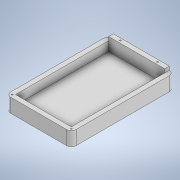
# Autodesk Inventor part: CARCASA SUPERIOR
Saved by Autodesk Inventor 2020 (Build 240168000, 168)
## iProperties
Created: 2022-05-22
Part Number: CARCASA SUPERIOR
Material: Generic
Document SubType Name: Modeling
Designer: juanc
Density: 1 g/cm^3
Appearance: Default
Author: juanc
## iProperties of the stored document _3DPrint.ipt
Created: 2022-05-23
Part Number: _3DPrint
Material: Generic
Document SubType Name: Modeling
Designer: juanc
Density: 1 g/cm^3
Appearance: Default
Author: juanc
Autodesk Inventor part; units mm, degrees
ref_plane "YZ Plane" through (0, 0, 0) normal (1, 0, 0) x (0, 1, 0)
ref_plane "XZ Plane" through (0, 0, 0) normal (0, 1, 0) x (-1, 0, 0)
ref_plane "XY Plane" through (0, 0, 0) normal (0, 0, 1) x (1, 0, 0)
sketch "Sketch1" plane through (0, 0, 0) normal (0, 1, 0) x (-1, 0, 0)
  line L0 (0, 0) -> (70, 0)
  line L1 (70, 0) -> (70, -110)
  line L2 (70, -110) -> (0, -110)
  line L3 (0, -110) -> (0, 0)
  line L4 (70, 0) -> (0, -110) construction
  line L5 (70, -110) -> (0, 0) construction
  line L6 (65, -5) -> (5, -5)
  line L7 (5, -5) -> (5, -105)
  line L8 (5, -105) -> (65, -105)
  line L9 (65, -105) -> (65, -5)
  line L10 (65, -5) -> (5, -105) construction
  line L11 (5, -5) -> (65, -105) construction
  point P0 (35, -55)
  dimension "d0" = 70
  dimension "d1" = 110
  dimension "d2" = 60
  dimension "d3" = 100
  constraints: 24 end point, 4 parallel, 3 midpoint, 2 horizontal, 2 perpendicular
  measures "d0" distance of L1.end L2.end
  measures "d1" distance of L0.end L1.end
  measures "d2" distance of L8.end L7.end
  measures "d3" distance of L7.end L6.end
extrude "Extrusion1" add sketch "Sketch1" along normal blind 15
extrude "Extrusion2" add sketch "Sketch1" along normal blind 5 contours L9 L8 L7 L6
fillet "Fillet1" radius 5 4 edges at (0, 7.5, -110) (0, 7.5, 0) (-70, 7.5, 0) (-70, 7.5, -110)
sketch "Sketch2" plane through (-5, 0, -110) normal (0, 0, -1) x (-1, 0, 0)
  line L0 (0, 15) -> (60, 15) projected
  line L1 (60, 15) -> (0, 15)
  line L2 (0, 15) -> (0, 19)
  line L3 (0, 19) -> (60, 19)
  line L4 (60, 19) -> (60, 15)
  point P0 (-5, 0)
  dimension "d9" = 60
  dimension "d10" = 4
  constraints: 8 end point, 2 parallel, 1 horizontal, 1 perpendicular
  measures "d9" distance of L2.end L3.end
  measures "d10" distance of L1.end L2.end
extrude "Extrusion3" add sketch "Sketch2" against normal blind 5
sketch "Sketch3" plane through (0, 0, 0) normal (0, -1, 0) x (1, 0, 0)
  arc A0 (-65, 0) -> (-70, -5) centre (-65, -5) ccw construction
  line L0 (-65, -5) -> (-66.7678, -3.2322) construction
  line L1 (-65, -5) -> (-62.5, -5) construction
  arc A1 (0, -5) -> (-5, 0) centre (-5, -5) ccw construction
  line L2 (-5, -5) -> (-3.2322, -3.2322) construction
  point P0 (0, 0)
  dimension "d13" = 2.5
  dimension "d14" = 135
  dimension "d15" = 2.5
  constraints: 6 end point, 2 coincident, 1 equal length, 1 horizontal
  measures "d13" distance of L0.start L0.end
  measures "d14" angle of L1 L0
  measures "d15" distance of L2.start L2.end
hole "Hole1" at (-66.7678, 0, -3.2322) at (-3.2322, 0, -3.2322) direction (0, 1, 0) diameter 1.5 depth 40 tip angle 118 counterbore diameter 2.5 counterbore depth 1
sketch "Sketch4" plane through (0, 0, 0) normal (0, -1, 0) x (1, 0, 0)
  line L0 (-65, -105) -> (-65, -110) construction
  line L1 (-5, -110) -> (-5, -105) construction
  line L2 (-5, -105) -> (-5, -5) construction
  line L3 (-5, -110) -> (-5, -105) construction
  line L4 (-5, -110) -> (-65, -110) construction
  line L5 (-35, -107.5) -> (-5, -107.5) construction
  line L6 (-35, -107.5) -> (-65, -107.5) construction
  line L7 (-35, -107.5) -> (-15, -107.5) construction
  line L8 (-35, -107.5) -> (-15, -107.5) construction
  line L9 (-35, -107.5) -> (-55, -107.5) construction
  line L10 (-35, -107.5) -> (-15, -107.5) construction
  point P0 (0, 0)
  dimension "d23" = 20
  dimension "d24" = 0
  dimension "d25" = 20
  dimension "d26" = 180
  constraints: 14 end point, 4 collinear, 2 coincident, 2 horizontal, 2 midpoint
  measures "d23" distance of L5.start L7.end
  measures "d24" distance between parallel lines of L7 L8
  measures "d25" distance of L5.start L9.end
  measures "d26" angle of L9 L10
hole "Hole2" at (-55, 0, -107.5) at (-15, 0, -107.5) direction (0, 1, 0) diameter 1.5 depth 40 tip angle 118 counterbore diameter 2.5 counterbore depth 1
sketch "Sketch5" plane through (0, 0, 0) normal (0, -1, 0) x (1, 0, 0)
  line L0 (-19.9406, -8.9451) -> (-19.9406, -100.011) construction
  line L1 (-19.9406, -100.011) -> (-26.1694, -100.011) construction
  line L2 (-26.1694, -100.011) -> (-26.1694, -8.9451) construction
  line L3 (-26.1694, -8.9451) -> (-19.9406, -8.9451) construction
  line L4 (-53.1117, -60.5446) -> (-53.1117, -96.1252) construction
  line L5 (-53.1117, -96.1252) -> (-61.1378, -96.1252) construction
  line L6 (-61.1378, -96.1252) -> (-61.1378, -60.5446) construction
  line L7 (-61.1378, -60.5446) -> (-53.1117, -60.5446) construction
  line L8 (-23.7466, -10.3806) -> (-26.0645, -10.3806)
  line L9 (-26.0645, -10.3806) -> (-26.0645, -9.5603)
  line L10 (-26.0645, -9.5603) -> (-20.0503, -9.5603)
  spline S0 degree 2 poles (-20.0503, -9.5603) (-20.0074, -10.4951) (-20.0074, -10.6859) knots 0 0 0 1 1 1
  spline S1 degree 2 poles (-20.0074, -10.6859) (-20.0074, -13.309) (-21.7625, -13.309) knots 0 0 0 1 1 1
  spline S2 degree 2 poles (-21.7625, -13.309) (-23.7895, -13.309) (-23.7895, -10.9911) knots 0 0 0 1 1 1
  spline S3 degree 2 poles (-23.7895, -10.9911) (-23.7895, -10.848) (-23.7466, -10.3806) knots 0 0 0 1 1 1
  line L11 (-20.7896, -10.3806) -> (-23.0073, -10.3806)
  spline S4 degree 2 poles (-23.0073, -10.3806) (-23.0502, -10.9053) (-23.0502, -10.9339) knots 0 0 0 1 1 1
  spline S5 degree 2 poles (-23.0502, -10.9339) (-23.0502, -12.4648) (-21.8484, -12.4648) knots 0 0 0 1 1 1
  spline S6 degree 2 poles (-21.8484, -12.4648) (-20.7466, -12.4648) (-20.7466, -10.829) knots 0 0 0 1 1 1
  spline S7 degree 2 poles (-20.7466, -10.829) (-20.7466, -10.6668) (-20.7896, -10.3806) knots 0 0 0 1 1 1
  line L12 (-26.0645, -17.5967) -> (-23.4795, -15.9894)
  spline S8 degree 2 poles (-23.4795, -15.9894) (-23.4795, -15.7128) (-23.4366, -15.1166) knots 0 0 0 1 1 1
  line L13 (-23.4366, -15.1166) -> (-26.0645, -15.1166)
  line L14 (-26.0645, -15.1166) -> (-26.0645, -14.2963)
  line L15 (-26.0645, -14.2963) -> (-20.0455, -14.2963)
  spline S9 degree 2 poles (-20.0455, -14.2963) (-20.0455, -14.3392) (-19.9835, -15.5268) (-19.9835, -15.7986) knots 0 0 0 1 2 2 2
  spline S10 degree 2 poles (-19.9835, -15.7986) (-19.9835, -17.9687) (-21.71, -17.9687) knots 0 0 0 1 1 1
  spline S11 degree 2 poles (-21.71, -17.9687) (-22.2776, -17.9687) (-23.1838, -17.2723) (-23.2935, -16.7906) knots 0 0 0 1 2 2 2
  line L16 (-23.2935, -16.7906) -> (-26.0645, -18.5362)
  line L17 (-26.0645, -18.5362) -> (-26.0645, -17.5967)
  line L18 (-20.7848, -15.1166) -> (-22.7402, -15.1166)
  spline S12 degree 2 poles (-22.7402, -15.1166) (-22.7831, -15.4123) (-22.7831, -15.6937) knots 0 0 0 1 1 1
  spline S13 degree 2 poles (-22.7831, -15.6937) (-22.7831, -16.4329) (-22.3062, -17.1054) (-21.691, -17.1054) knots 0 0 0 1 2 2 2
  spline S14 degree 2 poles (-21.691, -17.1054) (-21.1854, -17.1054) (-20.7419, -16.3805) (-20.7419, -15.6031) knots 0 0 0 1 2 2 2
  spline S15 degree 2 poles (-20.7419, -15.6031) (-20.7419, -15.4791) (-20.7848, -15.1166) knots 0 0 0 1 1 1
  spline S16 degree 2 poles (-23.0073, -18.8653) (-21.7005, -18.8653) (-19.9406, -20.1769) (-19.9406, -21.2881) knots 0 0 0 1 2 2 2
  spline S17 degree 2 poles (-19.9406, -21.2881) (-19.9406, -22.5425) (-21.5574, -23.8779) (-23.0073, -23.8779) knots 0 0 0 1 2 2 2
  spline S18 degree 2 poles (-23.0073, -23.8779) (-24.4906, -23.8779) (-26.1694, -22.5377) (-26.1694, -21.2881) knots 0 0 0 1 2 2 2
  spline S19 degree 2 poles (-26.1694, -21.2881) (-26.1694, -20.153) (-24.3952, -18.8653) (-23.0073, -18.8653) knots 0 0 0 1 2 2 2
  spline S20 degree 2 poles (-23.0073, -19.7286) (-24.0423, -19.7286) (-25.4301, -20.5441) (-25.4301, -21.2881) knots 0 0 0 1 2 2 2
  spline S21 degree 2 poles (-25.4301, -21.2881) (-25.4301, -22.1323) (-24.1567, -23.0146) (-23.0073, -23.0146) knots 0 0 0 1 2 2 2
  spline S22 degree 2 poles (-23.0073, -23.0146) (-20.6799, -23.0146) (-20.6799, -21.2881) knots 0 0 0 1 1 1
  spline S23 degree 2 poles (-20.6799, -21.2881) (-20.6799, -20.525) (-21.9294, -19.7286) (-23.0073, -19.7286) knots 0 0 0 1 2 2 2
  line L19 (-23.3698, -27.0209) -> (-26.0645, -27.0209)
  line L20 (-26.0645, -27.0209) -> (-26.0645, -26.2006)
  line L21 (-26.0645, -26.2006) -> (-23.3698, -26.2006)
  line L22 (-23.3698, -26.2006) -> (-20.0455, -24.2594)
  line L23 (-20.0455, -24.2594) -> (-20.0455, -25.1036)
  line L24 (-20.0455, -25.1036) -> (-22.6735, -26.606)
  line L25 (-22.6735, -26.606) -> (-20.0455, -28.1083)
  line L26 (-20.0455, -28.1083) -> (-20.0455, -28.9525)
  line L27 (-20.0455, -28.9525) -> (-23.3698, -27.0209)
  line L28 (-20.7848, -30.4405) -> (-22.4588, -30.4405)
  line L29 (-22.4588, -30.4405) -> (-22.4588, -32.3864)
  line L30 (-22.4588, -32.3864) -> (-23.1552, -32.3864)
  line L31 (-23.1552, -32.3864) -> (-23.1552, -30.4405)
  line L32 (-23.1552, -30.4405) -> (-25.3252, -30.4405)
  line L33 (-25.3252, -30.4405) -> (-25.3252, -33.1734)
  line L34 (-25.3252, -33.1734) -> (-26.0645, -33.1734)
  line L35 (-26.0645, -33.1734) -> (-26.0645, -29.6202)
  line L36 (-26.0645, -29.6202) -> (-20.0455, -29.6202)
  line L37 (-20.0455, -29.6202) -> (-20.0455, -33.1734)
  line L38 (-20.0455, -33.1734) -> (-20.7848, -33.1734)
  line L39 (-20.7848, -33.1734) -> (-20.7848, -30.4405)
  line L40 (-20.2697, -37.9666) -> (-20.9708, -37.6899)
  spline S24 degree 2 poles (-20.9708, -37.6899) (-20.6846, -37.2989) (-20.6846, -36.4547) knots 0 0 0 1 1 1
  spline S25 degree 2 poles (-20.6846, -36.4547) (-20.6846, -35.6582) (-22.0487, -34.7043) (-23.1265, -34.7043) knots 0 0 0 1 2 2 2
  spline S26 degree 2 poles (-23.1265, -34.7043) (-24.152, -34.7043) (-25.4301, -35.6868) (-25.4301, -36.4594) knots 0 0 0 1 2 2 2
  spline S27 degree 2 poles (-25.4301, -36.4594) (-25.4301, -37.3084) (-24.8292, -37.7615) knots 0 0 0 1 1 1
  line L41 (-24.8292, -37.7615) -> (-25.4588, -38.2146)
  spline S28 degree 2 poles (-25.4588, -38.2146) (-26.1694, -37.4992) (-26.1694, -36.3736) knots 0 0 0 1 1 1
  spline S29 degree 2 poles (-26.1694, -36.3736) (-26.1694, -35.1956) (-24.4667, -33.8411) (-23.0741, -33.8411) knots 0 0 0 1 2 2 2
  spline S30 degree 2 poles (-23.0741, -33.8411) (-21.7291, -33.8411) (-19.9454, -35.2862) (-19.9454, -36.4308) knots 0 0 0 1 2 2 2
  spline S31 degree 2 poles (-19.9454, -36.4308) (-19.9454, -37.4133) (-20.2697, -37.9666) knots 0 0 0 1 1 1
  line L42 (-20.7848, -41.3528) -> (-26.0645, -41.3528)
  line L43 (-26.0645, -41.3528) -> (-26.0645, -40.5325)
  line L44 (-26.0645, -40.5325) -> (-20.7848, -40.5325)
  line L45 (-20.7848, -40.5325) -> (-20.7848, -38.62)
  line L46 (-20.7848, -38.62) -> (-20.0455, -38.62)
  line L47 (-20.0455, -38.62) -> (-20.0455, -43.3512)
  line L48 (-20.0455, -43.3512) -> (-20.7848, -43.3512)
  line L49 (-20.7848, -43.3512) -> (-20.7848, -41.3528)
  spline S32 degree 2 poles (-23.0073, -43.7566) (-21.7005, -43.7566) (-19.9406, -45.0681) (-19.9406, -46.1794) knots 0 0 0 1 2 2 2
  spline S33 degree 2 poles (-19.9406, -46.1794) (-19.9406, -47.4337) (-21.5574, -48.7691) (-23.0073, -48.7691) knots 0 0 0 1 2 2 2
  spline S34 degree 2 poles (-23.0073, -48.7691) (-24.4906, -48.7691) (-26.1694, -47.429) (-26.1694, -46.1794) knots 0 0 0 1 2 2 2
  spline S35 degree 2 poles (-26.1694, -46.1794) (-26.1694, -45.0443) (-24.3952, -43.7566) (-23.0073, -43.7566) knots 0 0 0 1 2 2 2
  spline S36 degree 2 poles (-23.0073, -44.6198) (-24.0423, -44.6198) (-25.4301, -45.4354) (-25.4301, -46.1794) knots 0 0 0 1 2 2 2
  spline S37 degree 2 poles (-25.4301, -46.1794) (-25.4301, -47.0236) (-24.1567, -47.9059) (-23.0073, -47.9059) knots 0 0 0 1 2 2 2
  spline S38 degree 2 poles (-23.0073, -47.9059) (-20.6799, -47.9059) (-20.6799, -46.1794) knots 0 0 0 1 1 1
  spline S39 degree 2 poles (-20.6799, -46.1794) (-20.6799, -45.4163) (-21.9294, -44.6198) (-23.0073, -44.6198) knots 0 0 0 1 2 2 2
  line L50 (-26.0645, -52.3891) -> (-20.0455, -52.3891)
  line L51 (-20.0455, -52.3891) -> (-20.0455, -53.2094)
  line L52 (-20.0455, -53.2094) -> (-26.0645, -53.2094)
  line L53 (-26.0645, -53.2094) -> (-26.0645, -52.3891)
  line L54 (-26.1455, -58.4795) -> (-21.7482, -55.3699)
  line L55 (-21.7482, -55.3699) -> (-26.0645, -55.3699)
  line L56 (-26.0645, -55.3699) -> (-26.0645, -54.5877)
  line L57 (-26.0645, -54.5877) -> (-20.0455, -54.5877)
  line L58 (-20.0455, -54.5877) -> (-20.0455, -54.9168)
  line L59 (-20.0455, -54.9168) -> (-24.2044, -57.9454)
  line L60 (-24.2044, -57.9454) -> (-20.0455, -57.9454)
  line L61 (-20.0455, -57.9454) -> (-20.0455, -58.7275)
  line L62 (-20.0455, -58.7275) -> (-26.1455, -58.7275)
  line L63 (-26.1455, -58.7275) -> (-26.1455, -58.4795)
  line L64 (-20.7848, -62.1519) -> (-26.0645, -62.1519)
  line L65 (-26.0645, -62.1519) -> (-26.0645, -61.3316)
  line L66 (-26.0645, -61.3316) -> (-20.7848, -61.3316)
  line L67 (-20.7848, -61.3316) -> (-20.7848, -59.4191)
  line L68 (-20.7848, -59.4191) -> (-20.0455, -59.4191)
  line L69 (-20.0455, -59.4191) -> (-20.0455, -64.1503)
  line L70 (-20.0455, -64.1503) -> (-20.7848, -64.1503)
  line L71 (-20.7848, -64.1503) -> (-20.7848, -62.1519)
  line L72 (-20.7848, -65.6622) -> (-22.4588, -65.6622)
  line L73 (-22.4588, -65.6622) -> (-22.4588, -67.6081)
  line L74 (-22.4588, -67.6081) -> (-23.1552, -67.6081)
  line L75 (-23.1552, -67.6081) -> (-23.1552, -65.6622)
  line L76 (-23.1552, -65.6622) -> (-25.3252, -65.6622)
  line L77 (-25.3252, -65.6622) -> (-25.3252, -68.395)
  line L78 (-25.3252, -68.395) -> (-26.0645, -68.395)
  line L79 (-26.0645, -68.395) -> (-26.0645, -64.8419)
  line L80 (-26.0645, -64.8419) -> (-20.0455, -64.8419)
  line L81 (-20.0455, -64.8419) -> (-20.0455, -68.395)
  line L82 (-20.0455, -68.395) -> (-20.7848, -68.395)
  line L83 (-20.7848, -68.395) -> (-20.7848, -65.6622)
  line L84 (-20.4652, -73.5221) -> (-21.1425, -73.1787)
  spline S40 degree 2 poles (-21.1425, -73.1787) (-20.6846, -72.5587) (-20.6846, -71.9625) knots 0 0 0 1 1 1
  spline S41 degree 2 poles (-20.6846, -71.9625) (-20.6846, -71.0182) (-22.0153, -69.926) (-23.1122, -69.926) knots 0 0 0 1 2 2 2
  spline S42 degree 2 poles (-23.1122, -69.926) (-24.1567, -69.926) (-25.4301, -70.9991) (-25.4301, -71.9243) knots 0 0 0 1 2 2 2
  spline S43 degree 2 poles (-25.4301, -71.9243) (-25.4301, -72.5825) (-25.0343, -72.9879) knots 0 0 0 1 1 1
  line L85 (-25.0343, -72.9879) -> (-23.6226, -72.9879)
  line L86 (-23.6226, -72.9879) -> (-23.6226, -72.1533)
  line L87 (-23.6226, -72.1533) -> (-22.9262, -72.1533)
  line L88 (-22.9262, -72.1533) -> (-22.9262, -73.8082)
  line L89 (-22.9262, -73.8082) -> (-25.5494, -73.8082)
  spline S44 degree 2 poles (-25.5494, -73.8082) (-25.826, -73.4791) (-26.1694, -72.3059) (-26.1694, -71.7479) knots 0 0 0 1 2 2 2
  spline S45 degree 2 poles (-26.1694, -71.7479) (-26.1694, -70.5031) (-24.481, -69.0627) (-23.0788, -69.0627) knots 0 0 0 1 2 2 2
  spline S46 degree 2 poles (-23.0788, -69.0627) (-21.6814, -69.0627) (-19.9454, -70.6462) (-19.9454, -71.9911) knots 0 0 0 1 2 2 2
  spline S47 degree 2 poles (-19.9454, -71.9911) (-19.9454, -72.9307) (-20.4652, -73.5221) knots 0 0 0 1 1 1
  line L90 (-26.0645, -78.382) -> (-23.4795, -76.7748)
  spline S48 degree 2 poles (-23.4795, -76.7748) (-23.4795, -76.4981) (-23.4366, -75.902) knots 0 0 0 1 1 1
  line L91 (-23.4366, -75.902) -> (-26.0645, -75.902)
  line L92 (-26.0645, -75.902) -> (-26.0645, -75.0817)
  line L93 (-26.0645, -75.0817) -> (-20.0455, -75.0817)
  spline S49 degree 2 poles (-20.0455, -75.0817) (-20.0455, -75.1246) (-19.9835, -76.3121) (-19.9835, -76.584) knots 0 0 0 1 2 2 2
  spline S50 degree 2 poles (-19.9835, -76.584) (-19.9835, -78.7541) (-21.71, -78.7541) knots 0 0 0 1 1 1
  spline S51 degree 2 poles (-21.71, -78.7541) (-22.2776, -78.7541) (-23.1838, -78.0577) (-23.2935, -77.576) knots 0 0 0 1 2 2 2
  line L94 (-23.2935, -77.576) -> (-26.0645, -79.3216)
  line L95 (-26.0645, -79.3216) -> (-26.0645, -78.382)
  line L96 (-20.7848, -75.902) -> (-22.7402, -75.902)
  spline S52 degree 2 poles (-22.7402, -75.902) (-22.7831, -76.1977) (-22.7831, -76.4791) knots 0 0 0 1 1 1
  spline S53 degree 2 poles (-22.7831, -76.4791) (-22.7831, -77.2183) (-22.3062, -77.8908) (-21.691, -77.8908) knots 0 0 0 1 2 2 2
  spline S54 degree 2 poles (-21.691, -77.8908) (-21.1854, -77.8908) (-20.7419, -77.1659) (-20.7419, -76.3885) knots 0 0 0 1 2 2 2
  spline S55 degree 2 poles (-20.7419, -76.3885) (-20.7419, -76.2645) (-20.7848, -75.902) knots 0 0 0 1 1 1
  line L97 (-26.0645, -83.3565) -> (-24.7958, -82.9415)
  line L98 (-24.7958, -82.9415) -> (-24.7958, -80.7047)
  line L99 (-24.7958, -80.7047) -> (-26.0645, -80.2612)
  line L100 (-26.0645, -80.2612) -> (-26.0645, -79.3407)
  line L101 (-26.0645, -79.3407) -> (-19.9645, -81.7826)
  line L102 (-19.9645, -81.7826) -> (-19.9645, -82.002)
  line L103 (-19.9645, -82.002) -> (-26.0645, -84.2674)
  line L104 (-26.0645, -84.2674) -> (-26.0645, -83.3565)
  line L105 (-21.5431, -81.8541) -> (-24.1901, -80.9241)
  line L106 (-24.1901, -80.9241) -> (-24.1901, -82.7078)
  line L107 (-24.1901, -82.7078) -> (-21.5431, -81.8541)
  line L108 (-26.0645, -86.1084) -> (-26.0645, -84.897)
  line L109 (-26.0645, -84.897) -> (-20.0503, -84.897)
  spline S56 degree 2 poles (-20.0503, -84.897) (-20.0074, -86.0559) (-20.0074, -86.3802) knots 0 0 0 1 1 1
  spline S57 degree 2 poles (-20.0074, -86.3802) (-20.0074, -87.6394) (-21.5383, -89.1083) (-22.8118, -89.1083) knots 0 0 0 1 2 2 2
  spline S58 degree 2 poles (-22.8118, -89.1083) (-26.0645, -89.1083) (-26.0645, -86.1084) knots 0 0 0 1 1 1
  line L110 (-20.7896, -85.7173) -> (-25.2823, -85.7173)
  spline S59 degree 2 poles (-25.2823, -85.7173) (-25.3252, -85.9939) (-25.3252, -86.3993) knots 0 0 0 1 1 1
  spline S60 degree 2 poles (-25.3252, -86.3993) (-25.3252, -87.2626) (-24.0327, -88.2451) (-22.8833, -88.2451) knots 0 0 0 1 2 2 2
  spline S61 degree 2 poles (-22.8833, -88.2451) (-20.7466, -88.2451) (-20.7466, -86.3278) knots 0 0 0 1 1 1
  spline S62 degree 2 poles (-20.7466, -86.3278) (-20.7466, -86.2133) (-20.7896, -85.7173) knots 0 0 0 1 1 1
  spline S63 degree 2 poles (-23.0073, -89.7713) (-21.7005, -89.7713) (-19.9406, -91.0828) (-19.9406, -92.1941) knots 0 0 0 1 2 2 2
  spline S64 degree 2 poles (-19.9406, -92.1941) (-19.9406, -93.4484) (-21.5574, -94.7838) (-23.0073, -94.7838) knots 0 0 0 1 2 2 2
  spline S65 degree 2 poles (-23.0073, -94.7838) (-24.4906, -94.7838) (-26.1694, -93.4437) (-26.1694, -92.1941) knots 0 0 0 1 2 2 2
  spline S66 degree 2 poles (-26.1694, -92.1941) (-26.1694, -91.059) (-24.3952, -89.7713) (-23.0073, -89.7713) knots 0 0 0 1 2 2 2
  spline S67 degree 2 poles (-23.0073, -90.6345) (-24.0423, -90.6345) (-25.4301, -91.4501) (-25.4301, -92.1941) knots 0 0 0 1 2 2 2
  spline S68 degree 2 poles (-25.4301, -92.1941) (-25.4301, -93.0383) (-24.1567, -93.9206) (-23.0073, -93.9206) knots 0 0 0 1 2 2 2
  spline S69 degree 2 poles (-23.0073, -93.9206) (-20.6799, -93.9206) (-20.6799, -92.1941) knots 0 0 0 1 1 1
  spline S70 degree 2 poles (-20.6799, -92.1941) (-20.6799, -91.431) (-21.9294, -90.6345) (-23.0073, -90.6345) knots 0 0 0 1 2 2 2
  line L111 (-26.0645, -99.0715) -> (-23.4795, -97.4642)
  spline S71 degree 2 poles (-23.4795, -97.4642) (-23.4795, -97.1876) (-23.4366, -96.5914) knots 0 0 0 1 1 1
  line L112 (-23.4366, -96.5914) -> (-26.0645, -96.5914)
  line L113 (-26.0645, -96.5914) -> (-26.0645, -95.7711)
  line L114 (-26.0645, -95.7711) -> (-20.0455, -95.7711)
  spline S72 degree 2 poles (-20.0455, -95.7711) (-20.0455, -95.814) (-19.9835, -97.0016) (-19.9835, -97.2734) knots 0 0 0 1 2 2 2
  spline S73 degree 2 poles (-19.9835, -97.2734) (-19.9835, -99.4435) (-21.71, -99.4435) knots 0 0 0 1 1 1
  spline S74 degree 2 poles (-21.71, -99.4435) (-22.2776, -99.4435) (-23.1838, -98.7472) (-23.2935, -98.2655) knots 0 0 0 1 2 2 2
  line L115 (-23.2935, -98.2655) -> (-26.0645, -100.011)
  line L116 (-26.0645, -100.011) -> (-26.0645, -99.0715)
  line L117 (-20.7848, -96.5914) -> (-22.7402, -96.5914)
  spline S75 degree 2 poles (-22.7402, -96.5914) (-22.7831, -96.8871) (-22.7831, -97.1685) knots 0 0 0 1 1 1
  spline S76 degree 2 poles (-22.7831, -97.1685) (-22.7831, -97.9078) (-22.3062, -98.5802) (-21.691, -98.5802) knots 0 0 0 1 2 2 2
  spline S77 degree 2 poles (-21.691, -98.5802) (-21.1854, -98.5802) (-20.7419, -97.8553) (-20.7419, -97.0779) knots 0 0 0 1 2 2 2
  spline S78 degree 2 poles (-20.7419, -97.0779) (-20.7419, -96.9539) (-20.7848, -96.5914) knots 0 0 0 1 1 1
  line L118 (-56.224, -63.0344) -> (-56.224, -62.5799)
  line L119 (-56.224, -62.5799) -> (-53.5959, -61.2313)
  line L120 (-53.5959, -61.2313) -> (-56.224, -61.2313)
  line L121 (-56.224, -61.2313) -> (-56.224, -60.8533)
  line L122 (-56.224, -60.8533) -> (-53.176, -60.8533)
  line L123 (-53.176, -60.8533) -> (-53.176, -61.4289)
  line L124 (-53.176, -61.4289) -> (-55.5892, -62.6565)
  line L125 (-55.5892, -62.6565) -> (-53.176, -62.6565)
  line L126 (-53.176, -62.6565) -> (-53.176, -63.0344)
  line L127 (-53.176, -63.0344) -> (-56.224, -63.0344)
  spline S79 degree 2 poles (-53.5242, -65.8082) (-53.7268, -65.9811) (-54.3196, -66.1738) (-54.7, -66.1738) knots 0 0 0 1 2 2 2
  spline S80 degree 2 poles (-54.7, -66.1738) (-55.0705, -66.1738) (-55.6707, -65.986) (-55.8732, -65.8082) knots 0 0 0 1 2 2 2
  spline S81 degree 2 poles (-55.8732, -65.8082) (-56.0856, -65.6205) (-56.2882, -65.124) (-56.2882, -64.8251) knots 0 0 0 1 2 2 2
  spline S82 degree 2 poles (-56.2882, -64.8251) (-56.2882, -64.5164) (-56.0782, -64.0224) (-55.8732, -63.8421) knots 0 0 0 1 2 2 2
  spline S83 degree 2 poles (-55.8732, -63.8421) (-55.6707, -63.6667) (-55.0754, -63.479) (-54.7, -63.479) knots 0 0 0 1 2 2 2
  spline S84 degree 2 poles (-54.7, -63.479) (-54.3171, -63.479) (-53.7342, -63.6692) (-53.5242, -63.8445) knots 0 0 0 1 2 2 2
  spline S85 degree 2 poles (-53.5242, -63.8445) (-53.3217, -64.0224) (-53.1117, -64.5189) (-53.1117, -64.8251) knots 0 0 0 1 2 2 2
  spline S86 degree 2 poles (-53.1117, -64.8251) (-53.1117, -65.1364) (-53.3291, -65.6353) (-53.5242, -65.8082) knots 0 0 0 1 2 2 2
  spline S87 degree 2 poles (-54.7, -65.7514) (-54.3986, -65.7514) (-53.9318, -65.6205) (-53.7786, -65.5019) knots 0 0 0 1 2 2 2
  spline S88 degree 2 poles (-53.7786, -65.5019) (-53.6206, -65.3809) (-53.4625, -65.04) (-53.4625, -64.8276) knots 0 0 0 1 2 2 2
  spline S89 degree 2 poles (-53.4625, -64.8276) (-53.4625, -64.6078) (-53.6156, -64.2768) (-53.7786, -64.1508) knots 0 0 0 1 2 2 2
  spline S90 degree 2 poles (-53.7786, -64.1508) (-53.9343, -64.0298) (-54.4036, -63.9013) (-54.7, -63.9013) knots 0 0 0 1 2 2 2
  spline S91 degree 2 poles (-54.7, -63.9013) (-55.3002, -63.9013) (-55.9374, -64.4052) (-55.9374, -64.8276) knots 0 0 0 1 2 2 2
  spline S92 degree 2 poles (-55.9374, -64.8276) (-55.9374, -65.25) (-55.3002, -65.7514) (-54.7, -65.7514) knots 0 0 0 1 2 2 2
  line L128 (-53.176, -68.7525) -> (-54.8753, -67.7225)
  line L129 (-54.8753, -67.7225) -> (-56.224, -67.7225)
  line L130 (-56.224, -67.7225) -> (-56.224, -67.3174)
  line L131 (-56.224, -67.3174) -> (-54.9173, -67.3174)
  line L132 (-54.9173, -67.3174) -> (-53.176, -66.2874)
  line L133 (-53.176, -66.2874) -> (-53.176, -66.7369)
  line L134 (-53.176, -66.7369) -> (-54.5172, -67.5224)
  line L135 (-54.5172, -67.5224) -> (-53.176, -68.3227)
  line L136 (-53.176, -68.3227) -> (-53.176, -68.7525)
  line L137 (-56.224, -68.7055) -> (-53.176, -69.7331)
  line L138 (-53.176, -69.7331) -> (-53.176, -70.232)
  line L139 (-53.176, -70.232) -> (-56.224, -71.2595)
  line L140 (-56.224, -71.2595) -> (-56.224, -70.8322)
  line L141 (-56.224, -70.8322) -> (-55.3718, -70.5556)
  line L142 (-55.3718, -70.5556) -> (-55.3718, -69.3922)
  line L143 (-55.3718, -69.3922) -> (-56.224, -69.1156)
  line L144 (-56.224, -69.1156) -> (-56.224, -68.7055)
  line L145 (-55.026, -70.4444) -> (-53.5909, -69.9726)
  line L146 (-53.5909, -69.9726) -> (-55.026, -69.5033)
  line L147 (-55.026, -69.5033) -> (-55.026, -70.4444)
  line L148 (-55.0754, -73.8876) -> (-55.0754, -72.7341)
  line L149 (-55.0754, -72.7341) -> (-54.7049, -72.7341)
  line L150 (-54.7049, -72.7341) -> (-54.7049, -73.8876)
  line L151 (-54.7049, -73.8876) -> (-55.0754, -73.8876)
  line L152 (-56.224, -75.3598) -> (-53.176, -76.3873)
  line L153 (-53.176, -76.3873) -> (-53.176, -76.8862)
  line L154 (-53.176, -76.8862) -> (-56.224, -77.9137)
  line L155 (-56.224, -77.9137) -> (-56.224, -77.4864)
  line L156 (-56.224, -77.4864) -> (-55.3718, -77.2098)
  line L157 (-55.3718, -77.2098) -> (-55.3718, -76.0464)
  line L158 (-55.3718, -76.0464) -> (-56.224, -75.7698)
  line L159 (-56.224, -75.7698) -> (-56.224, -75.3598)
  line L160 (-55.026, -77.0986) -> (-53.5909, -76.6269)
  line L161 (-53.5909, -76.6269) -> (-55.026, -76.1576)
  line L162 (-55.026, -76.1576) -> (-55.026, -77.0986)
  line L163 (-56.224, -79.9688) -> (-56.224, -78.2027)
  line L164 (-56.224, -78.2027) -> (-53.176, -78.2027)
  line L165 (-53.176, -78.2027) -> (-53.176, -78.6078)
  line L166 (-53.176, -78.6078) -> (-55.8633, -78.6078)
  line L167 (-55.8633, -78.6078) -> (-55.8633, -79.9688)
  line L168 (-55.8633, -79.9688) -> (-56.224, -79.9688)
  spline S93 degree 2 poles (-55.2878, -82.3548) (-55.5151, -82.3548) (-55.8633, -82.1819) (-55.977, -82.0387) knots 0 0 0 1 2 2 2
  spline S94 degree 2 poles (-55.977, -82.0387) (-56.1103, -81.8658) (-56.224, -81.473) (-56.224, -81.1618) knots 0 0 0 1 2 2 2
  line L169 (-56.224, -81.1618) -> (-56.224, -80.2874)
  line L170 (-56.224, -80.2874) -> (-53.176, -80.2874)
  line L171 (-53.176, -80.2874) -> (-53.176, -81.0951)
  spline S95 degree 2 poles (-53.176, -81.0951) (-53.176, -81.4212) (-53.218, -81.7472) (-53.2995, -81.8954) knots 0 0 0 1 2 2 2
  spline S96 degree 2 poles (-53.2995, -81.8954) (-53.3859, -82.0609) (-53.67, -82.2116) (-53.8626, -82.2116) knots 0 0 0 1 2 2 2
  spline S97 degree 2 poles (-53.8626, -82.2116) (-54.0775, -82.2116) (-54.4184, -81.9843) (-54.5147, -81.7843) knots 0 0 0 1 2 2 2
  line L172 (-54.5147, -81.7843) -> (-54.5295, -81.7843)
  spline S98 degree 2 poles (-54.5295, -81.7843) (-54.6036, -82.056) (-54.9964, -82.3548) (-55.2878, -82.3548) knots 0 0 0 1 2 2 2
  spline S99 degree 2 poles (-55.3051, -81.9325) (-55.1322, -81.9325) (-54.9099, -81.8337) (-54.8309, -81.6855) knots 0 0 0 1 2 2 2
  spline S100 degree 2 poles (-54.8309, -81.6855) (-54.7815, -81.5891) (-54.7518, -81.3619) (-54.7518, -81.1519) knots 0 0 0 1 2 2 2
  line L173 (-54.7518, -81.1519) -> (-54.7518, -80.6925)
  line L174 (-54.7518, -80.6925) -> (-55.8782, -80.6925)
  line L175 (-55.8782, -80.6925) -> (-55.8782, -81.021)
  spline S101 degree 2 poles (-55.8782, -81.021) (-55.8782, -81.2878) (-55.8288, -81.5941) (-55.7497, -81.7126) knots 0 0 0 1 2 2 2
  spline S102 degree 2 poles (-55.7497, -81.7126) (-55.6682, -81.8263) (-55.4657, -81.9325) (-55.3051, -81.9325) knots 0 0 0 1 2 2 2
  spline S103 degree 2 poles (-53.9194, -81.7892) (-53.8108, -81.7892) (-53.6477, -81.7151) (-53.6008, -81.6336) knots 0 0 0 1 2 2 2
  spline S104 degree 2 poles (-53.6008, -81.6336) (-53.5465, -81.5348) (-53.5218, -81.2952) (-53.5218, -81.0803) knots 0 0 0 1 2 2 2
  line L176 (-53.5218, -81.0803) -> (-53.5218, -80.6925)
  line L177 (-53.5218, -80.6925) -> (-54.4134, -80.6925)
  line L178 (-54.4134, -80.6925) -> (-54.4134, -81.1519)
  spline S105 degree 2 poles (-54.4134, -81.1519) (-54.4134, -81.3421) (-54.3739, -81.5224) (-54.3122, -81.6188) knots 0 0 0 1 2 2 2
  spline S106 degree 2 poles (-54.3122, -81.6188) (-54.2529, -81.7126) (-54.0627, -81.7892) (-53.9194, -81.7892) knots 0 0 0 1 2 2 2
  spline S107 degree 2 poles (-53.5242, -84.9138) (-53.7268, -85.0867) (-54.3196, -85.2793) (-54.7, -85.2793) knots 0 0 0 1 2 2 2
  spline S108 degree 2 poles (-54.7, -85.2793) (-55.0705, -85.2793) (-55.6707, -85.0916) (-55.8732, -84.9138) knots 0 0 0 1 2 2 2
  spline S109 degree 2 poles (-55.8732, -84.9138) (-56.0856, -84.7261) (-56.2882, -84.2296) (-56.2882, -83.9307) knots 0 0 0 1 2 2 2
  spline S110 degree 2 poles (-56.2882, -83.9307) (-56.2882, -83.622) (-56.0782, -83.128) (-55.8732, -82.9476) knots 0 0 0 1 2 2 2
  spline S111 degree 2 poles (-55.8732, -82.9476) (-55.6707, -82.7723) (-55.0754, -82.5846) (-54.7, -82.5846) knots 0 0 0 1 2 2 2
  spline S112 degree 2 poles (-54.7, -82.5846) (-54.3171, -82.5846) (-53.7342, -82.7747) (-53.5242, -82.9501) knots 0 0 0 1 2 2 2
  spline S113 degree 2 poles (-53.5242, -82.9501) (-53.3217, -83.128) (-53.1117, -83.6244) (-53.1117, -83.9307) knots 0 0 0 1 2 2 2
  spline S114 degree 2 poles (-53.1117, -83.9307) (-53.1117, -84.2419) (-53.3291, -84.7409) (-53.5242, -84.9138) knots 0 0 0 1 2 2 2
  spline S115 degree 2 poles (-54.7, -84.857) (-54.3986, -84.857) (-53.9318, -84.7261) (-53.7786, -84.6075) knots 0 0 0 1 2 2 2
  spline S116 degree 2 poles (-53.7786, -84.6075) (-53.6206, -84.4865) (-53.4625, -84.1456) (-53.4625, -83.9332) knots 0 0 0 1 2 2 2
  spline S117 degree 2 poles (-53.4625, -83.9332) (-53.4625, -83.7133) (-53.6156, -83.3824) (-53.7786, -83.2564) knots 0 0 0 1 2 2 2
  spline S118 degree 2 poles (-53.7786, -83.2564) (-53.9343, -83.1354) (-54.4036, -83.0069) (-54.7, -83.0069) knots 0 0 0 1 2 2 2
  spline S119 degree 2 poles (-54.7, -83.0069) (-55.3002, -83.0069) (-55.9374, -83.5108) (-55.9374, -83.9332) knots 0 0 0 1 2 2 2
  spline S120 degree 2 poles (-55.9374, -83.9332) (-55.9374, -84.3556) (-55.3002, -84.857) (-54.7, -84.857) knots 0 0 0 1 2 2 2
  line L179 (-56.224, -88.0828) -> (-56.224, -87.5567)
  line L180 (-56.224, -87.5567) -> (-55.0112, -86.5934)
  line L181 (-55.0112, -86.5934) -> (-55.0112, -86.129)
  line L182 (-55.0112, -86.129) -> (-56.224, -86.129)
  line L183 (-56.224, -86.129) -> (-56.224, -85.7239)
  line L184 (-56.224, -85.7239) -> (-53.176, -85.7239)
  line L185 (-53.176, -85.7239) -> (-53.176, -86.5094)
  spline S121 degree 2 poles (-53.176, -86.5094) (-53.176, -86.7712) (-53.2328, -87.1244) (-53.3365, -87.285) knots 0 0 0 1 2 2 2
  spline S122 degree 2 poles (-53.3365, -87.285) (-53.4403, -87.4455) (-53.7638, -87.6308) (-54.0034, -87.6308) knots 0 0 0 1 2 2 2
  spline S123 degree 2 poles (-54.0034, -87.6308) (-54.3369, -87.6308) (-54.7889, -87.2899) (-54.8976, -86.9985) knots 0 0 0 1 2 2 2
  line L186 (-54.8976, -86.9985) -> (-56.224, -88.0828)
  spline S124 degree 2 poles (-54.0355, -87.2084) (-53.9021, -87.2084) (-53.6971, -87.1146) (-53.6304, -87.0158) knots 0 0 0 1 2 2 2
  spline S125 degree 2 poles (-53.6304, -87.0158) (-53.5736, -86.9293) (-53.5267, -86.6996) (-53.5267, -86.5316) knots 0 0 0 1 2 2 2
  line L187 (-53.5267, -86.5316) -> (-53.5267, -86.129)
  line L188 (-53.5267, -86.129) -> (-54.6728, -86.129)
  line L189 (-54.6728, -86.129) -> (-54.6728, -86.4847)
  spline S126 degree 2 poles (-54.6728, -86.4847) (-54.6728, -86.6601) (-54.611, -86.9392) (-54.5147, -87.0355) knots 0 0 0 1 2 2 2
  spline S127 degree 2 poles (-54.5147, -87.0355) (-54.4307, -87.1244) (-54.1936, -87.2084) (-54.0355, -87.2084) knots 0 0 0 1 2 2 2
  line L190 (-56.224, -90.5059) -> (-56.224, -90.0514)
  line L191 (-56.224, -90.0514) -> (-53.5959, -88.7028)
  line L192 (-53.5959, -88.7028) -> (-56.224, -88.7028)
  line L193 (-56.224, -88.7028) -> (-56.224, -88.3249)
  line L194 (-56.224, -88.3249) -> (-53.176, -88.3249)
  line L195 (-53.176, -88.3249) -> (-53.176, -88.9004)
  line L196 (-53.176, -88.9004) -> (-55.5892, -90.128)
  line L197 (-55.5892, -90.128) -> (-53.176, -90.128)
  line L198 (-53.176, -90.128) -> (-53.176, -90.5059)
  line L199 (-53.176, -90.5059) -> (-56.224, -90.5059)
  spline S128 degree 2 poles (-53.5242, -93.2797) (-53.7268, -93.4526) (-54.3196, -93.6453) (-54.7, -93.6453) knots 0 0 0 1 2 2 2
  spline S129 degree 2 poles (-54.7, -93.6453) (-55.0705, -93.6453) (-55.6707, -93.4576) (-55.8732, -93.2797) knots 0 0 0 1 2 2 2
  spline S130 degree 2 poles (-55.8732, -93.2797) (-56.0856, -93.092) (-56.2882, -92.5955) (-56.2882, -92.2967) knots 0 0 0 1 2 2 2
  spline S131 degree 2 poles (-56.2882, -92.2967) (-56.2882, -91.9879) (-56.0782, -91.4939) (-55.8732, -91.3136) knots 0 0 0 1 2 2 2
  spline S132 degree 2 poles (-55.8732, -91.3136) (-55.6707, -91.1382) (-55.0754, -90.9505) (-54.7, -90.9505) knots 0 0 0 1 2 2 2
  spline S133 degree 2 poles (-54.7, -90.9505) (-54.3171, -90.9505) (-53.7342, -91.1407) (-53.5242, -91.3161) knots 0 0 0 1 2 2 2
  spline S134 degree 2 poles (-53.5242, -91.3161) (-53.3217, -91.4939) (-53.1117, -91.9904) (-53.1117, -92.2967) knots 0 0 0 1 2 2 2
  spline S135 degree 2 poles (-53.1117, -92.2967) (-53.1117, -92.6079) (-53.3291, -93.1068) (-53.5242, -93.2797) knots 0 0 0 1 2 2 2
  spline S136 degree 2 poles (-54.7, -93.2229) (-54.3986, -93.2229) (-53.9318, -93.092) (-53.7786, -92.9734) knots 0 0 0 1 2 2 2
  spline S137 degree 2 poles (-53.7786, -92.9734) (-53.6206, -92.8524) (-53.4625, -92.5115) (-53.4625, -92.2991) knots 0 0 0 1 2 2 2
  spline S138 degree 2 poles (-53.4625, -92.2991) (-53.4625, -92.0793) (-53.6156, -91.7483) (-53.7786, -91.6223) knots 0 0 0 1 2 2 2
  spline S139 degree 2 poles (-53.7786, -91.6223) (-53.9343, -91.5013) (-54.4036, -91.3729) (-54.7, -91.3729) knots 0 0 0 1 2 2 2
  spline S140 degree 2 poles (-54.7, -91.3729) (-55.3002, -91.3729) (-55.9374, -91.8768) (-55.9374, -92.2991) knots 0 0 0 1 2 2 2
  spline S141 degree 2 poles (-55.9374, -92.2991) (-55.9374, -92.7215) (-55.3002, -93.2229) (-54.7, -93.2229) knots 0 0 0 1 2 2 2
  line L200 (-56.224, -96.0338) -> (-56.224, -93.9046)
  line L201 (-56.224, -93.9046) -> (-55.8461, -93.9046)
  line L202 (-55.8461, -93.9046) -> (-53.5366, -95.5348)
  line L203 (-53.5366, -95.5348) -> (-53.5366, -93.9787)
  line L204 (-53.5366, -93.9787) -> (-53.176, -93.9787)
  line L205 (-53.176, -93.9787) -> (-53.176, -95.9918)
  line L206 (-53.176, -95.9918) -> (-53.5415, -95.9918)
  line L207 (-53.5415, -95.9918) -> (-55.8633, -94.3443)
  line L208 (-55.8633, -94.3443) -> (-55.8633, -96.0338)
  line L209 (-55.8633, -96.0338) -> (-56.224, -96.0338)
  point P0 (0, 0)
  constraints: 4 other
emboss "Emboss1" sketch "Sketch5" operation cut depth 1 direction (0, 1, 0)
sketch "Sketch7" plane through (0, 0, 0) normal (0, -1, 0) x (1, 0, 0)
  line L0 (-53.1072, -10.97) -> (-53.1072, -34.781) construction
  line L1 (-53.1072, -34.781) -> (-57.1555, -34.781) construction
  line L2 (-57.1555, -34.781) -> (-57.1555, -10.97) construction
  line L3 (-57.1555, -10.97) -> (-53.1072, -10.97) construction
  line L4 (-56.1552, -12.3409) -> (-56.1552, -11.1602)
  line L5 (-56.1552, -11.1602) -> (-55.8439, -11.1602)
  line L6 (-55.8439, -11.1602) -> (-55.8439, -11.548)
  line L7 (-55.8439, -11.548) -> (-53.4184, -11.548)
  line L8 (-53.4184, -11.548) -> (-53.4184, -11.1602)
  line L9 (-53.4184, -11.1602) -> (-53.1072, -11.1602)
  line L10 (-53.1072, -11.1602) -> (-53.1072, -12.3409)
  line L11 (-53.1072, -12.3409) -> (-53.4184, -12.3409)
  line L12 (-53.4184, -12.3409) -> (-53.4184, -11.9531)
  line L13 (-53.4184, -11.9531) -> (-55.8439, -11.9531)
  line L14 (-55.8439, -11.9531) -> (-55.8439, -12.3409)
  line L15 (-55.8439, -12.3409) -> (-56.1552, -12.3409)
  spline S0 degree 2 poles (-55.219, -14.9097) (-55.4463, -14.9097) (-55.7945, -14.7368) (-55.9082, -14.5935) knots 0 0 0 1 2 2 2
  spline S1 degree 2 poles (-55.9082, -14.5935) (-56.0415, -14.4206) (-56.1552, -14.0279) (-56.1552, -13.7167) knots 0 0 0 1 2 2 2
  line L16 (-56.1552, -13.7167) -> (-56.1552, -12.8423)
  line L17 (-56.1552, -12.8423) -> (-53.1072, -12.8423)
  line L18 (-53.1072, -12.8423) -> (-53.1072, -13.65)
  spline S2 degree 2 poles (-53.1072, -13.65) (-53.1072, -13.976) (-53.1491, -14.3021) (-53.2307, -14.4503) knots 0 0 0 1 2 2 2
  spline S3 degree 2 poles (-53.2307, -14.4503) (-53.3171, -14.6158) (-53.6012, -14.7664) (-53.7938, -14.7664) knots 0 0 0 1 2 2 2
  spline S4 degree 2 poles (-53.7938, -14.7664) (-54.0087, -14.7664) (-54.3496, -14.5392) (-54.4459, -14.3391) knots 0 0 0 1 2 2 2
  line L19 (-54.4459, -14.3391) -> (-54.4607, -14.3391)
  spline S5 degree 2 poles (-54.4607, -14.3391) (-54.5348, -14.6108) (-54.9276, -14.9097) (-55.219, -14.9097) knots 0 0 0 1 2 2 2
  spline S6 degree 2 poles (-55.2363, -14.4873) (-55.0634, -14.4873) (-54.8411, -14.3885) (-54.7621, -14.2403) knots 0 0 0 1 2 2 2
  spline S7 degree 2 poles (-54.7621, -14.2403) (-54.7127, -14.144) (-54.683, -13.9167) (-54.683, -13.7068) knots 0 0 0 1 2 2 2
  line L20 (-54.683, -13.7068) -> (-54.683, -13.2474)
  line L21 (-54.683, -13.2474) -> (-55.8094, -13.2474)
  line L22 (-55.8094, -13.2474) -> (-55.8094, -13.5759)
  spline S8 degree 2 poles (-55.8094, -13.5759) (-55.8094, -13.8426) (-55.76, -14.1489) (-55.6809, -14.2675) knots 0 0 0 1 2 2 2
  spline S9 degree 2 poles (-55.6809, -14.2675) (-55.5994, -14.3811) (-55.3969, -14.4873) (-55.2363, -14.4873) knots 0 0 0 1 2 2 2
  spline S10 degree 2 poles (-53.8506, -14.3441) (-53.742, -14.3441) (-53.5789, -14.27) (-53.532, -14.1884) knots 0 0 0 1 2 2 2
  spline S11 degree 2 poles (-53.532, -14.1884) (-53.4777, -14.0896) (-53.453, -13.85) (-53.453, -13.6352) knots 0 0 0 1 2 2 2
  line L23 (-53.453, -13.6352) -> (-53.453, -13.2474)
  line L24 (-53.453, -13.2474) -> (-54.3446, -13.2474)
  line L25 (-54.3446, -13.2474) -> (-54.3446, -13.7068)
  spline S12 degree 2 poles (-54.3446, -13.7068) (-54.3446, -13.897) (-54.3051, -14.0773) (-54.2434, -14.1736) knots 0 0 0 1 2 2 2
  spline S13 degree 2 poles (-54.2434, -14.1736) (-54.1841, -14.2675) (-53.9939, -14.3441) (-53.8506, -14.3441) knots 0 0 0 1 2 2 2
  point P0 (0, 0)
  constraints: 2 other
emboss "Emboss2" sketch "Sketch7" operation add depth 0.5 direction (0, 1, 0)
sketch "Sketch8" plane through (0, 0, 0) normal (0, -1, 0) x (1, 0, 0)
  point P0 (0, 0)
body "Solid1"
